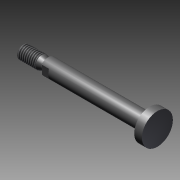
# Autodesk Inventor part: 536203 ADN-15-P-A_(KS)
Saved by Autodesk Inventor 2011 SP1 (Build 150282100, 282)
## iProperties
Created: 2018-05-28
Part Number: 536203 ADN-15-P-A_(KS)
Catalog Web Link: www.cadenas.de
Description: ADN-(KS)-Compact cylinder - piston rod
Vendor: FESTO
Document SubType Name: Modeling
Designer: psAdmin
Manufacturer: FESTO
Mass: 1.6217 g
Surface Area: 12.2965 cm^2
Volume: 1.6217 cm^3
Density: 1 g/cm^3
Category: PARTsolutions
Company: FESTO
Title: 536203 ADN-15-P-A_(KS)
Author: Cadenas PARTsolutions
Comments: Compact cylinder - piston rod
PSOL_IDENT_0: {$CADENAS_DATA\23d-libs\festo\parts\a\adn\parts\adn_ks.prj},229 {VTYP=3D},{NB=536203 ADN-15-P-A_(KS)
PSOL_IDENT_1: },{LINA=536203 ADN-15-P-A_(KS)},{NN=ADN-(KS)},{DATE=06.10.2015 11:54:02},{GEOMDATE=23.09.2015 12:10:
PSOL_IDENT_2: 00},{VERSION=},{LINEID=5510},{LINESUBID=-1},{WBVAR=DF,HUB,TH,Q,S2S20,K2,K5,K8,K10,S1,TT,R8}  {NB=536
PSOL_IDENT_3: 203 ADN-15-P-A_(KS)},{LINA=536203 ADN-15-P-A_(KS)},{KT=536203},{TNR=536203},{AUSF=ADN},{DF=P},{GA=A}
PSOL_IDENT_4: ,{WHX=4.2},{WH0=4.200},{WH1=0.000},{WH2=0.000},{WH3=0.000},{WHX1=4.2},{WHX2=4.75},{WH=4.2},{ZM=44.50
PSOL_IDENT_5: 0},{ZM2=0.000},{ZB=39.200},{ZB1=0.000},{ZB2=0.000},{ZB6=0.000},{ZA=35.000},{KDM=12},{HUBP=-},{HUB=15
PSOL_IDENT_6: },{HUB1=[1-300]},{HUB2=0},{HUB3=0},{HUB4=0},{TH=A},{THC='A','I'},{Q=-},{VAR1C='-','Q'},{S2S20=-},{VA
PSOL_IDENT_7: R2C='-','S2'},{VAR22C='-','S2'},{VAR222C='-','S2'},{K2=0},{VAR3C=0,[1-10]},{VAR33C=0,[1-10]},{K5=-},
PSOL_IDENT_8: {K5A='-','M6'},{K5I='-'},{K5S1A='-'},{K5S1I='-'},{K5C='-','M6'},{K5N=0},{K5P=0},{K5T=},{K8=0},{K10=-
PSOL_IDENT_9: },{K10A='-'},{K10N=},{S1=-},{TT=-},{TT1='-'},{R8=-},{R81='-'},{VAR4C=0,[1-300]},{VAR5C='-','S6'},{VA
PSOL_IDENT_10: R6C='-'},{VAR66C='-'},{VAR7C='-','R3'},{HUBALG=[1-300]},{A=10.000},{A1=0.000},{AF=8.000},{AF1=0.000}
PSOL_IDENT_11: ,{AF2=8.000},{AF3=0.000},{AF5=0.000},{AF7=0.000},{D8=0.000},{D9=0.000},{KF=M3},{KFN=3.000},{KF1=-},{
PSOL_IDENT_12: KF1C=0.0000},{KF2=-},{KF2C=0.0000},{KF3=M3},{KF3C=3.0000},{KF5=-},{KF5N=0},{KF7=-},{KF7N=0},{KK=M5},
PSOL_IDENT_13: {KKN=5},{KKP=0.80},{KK1=-},{KK1N=0.0000},{KK1P=0.00},{L2=35.000},{L8=0.000},{MM=6.000},{MM1=0.000},{
PSOL_IDENT_14: PL=6.000},{SF=5},{SF1=0},{SF3=5.5},{WL=2.700},{WL1=0.000},{QN=},{S2N=},{S1N=},{K2N=},{K8N=},{KKC3=3.
PSOL_IDENT_15: 800},{KKF2=0.400},{KKD5=0.900},{KKE2=20.000},{K5C3=0},{K5F2=0},{K5D5=0},{KK1C3=0.000},{KK1F2=0.000},
PSOL_IDENT_16: {KK1D5=0.000},{KK1E2=0.000},{L100S1=0.000},{L101S1=0.000},{L102S1=0.000},{L103S1=0.000},{D100S1=0.00
PSOL_IDENT_17: 0},{L100=0.400},{L101=1.500},{L102=8.000},{L103=11.000},{D100=3.300},{L100Q=0.400},{L101Q=1.500},{L1
PSOL_IDENT_18: 01K5=1.500},{L102Q=8.000},{L103Q=11.000},{D100Q=3.300},{L100S1K5=0.000},{L101S1K5=0.000},{L102S1K5=0
PSOL_IDENT_19: .000},{L103S1K5=0.000},{D100S1K5=0.000},{VERS=1},{TTN=},{R8N=},{D20=0.000},{XF31=3.000},{B31=2.700},
PSOL_IDENT_20: {DFALG='P'}
NN: ADN-(KS)
NT: Compact cylinder - piston rod
NB: 536203 ADN-15-P-A_(KS)
NBSYN: $TNR. $AUSF.-$HUB.-$DF.-$TH.$QN.$S2N.$K2N.$K5T.$K8N.$K10N.$S1N.$TTN.$R8N._(KS)
LINA: 536203 ADN-15-P-A_(KS)
TNR: 536203
AUSF: ADN
DF: P
GA: A
WHX: 4.200
WH0: 4.200
WH1: 0.000
WH2: 0.000
WH3: 0.000
WHX1: 4.200
WHX2: 4.750
WH: 4.200
ZM: 44.500
ZM2: 0.000
ZB: 39.200
ZB1: 0.000
ZB2: 0.000
ZB6: 0.000
ZA: 35.000
KDM: 12
HUBP: -
HUB: 15
TH: A
Q: -
S2S20: -
K2: 0
K5: -
K8: 0
K10: -
S1: -
TT: -
R8: -
A: 10.000
A1: 0.000
AF: 8.000
AF1: 0.000
AF2: 8.000
AF3: 0.000
AF5: 0.000
AF7: 0.000
D8: 0.000
D9: 0.000
KF: M3
KF1: -
KF2: -
KF3: M3
KF5: -
KF7: -
KK: M5
KK1: -
L2: 35.000
L8: 0.000
MM: 6.000
MM1: 0.000
PL: 6.000
SF: 5
SF1: 0
SF3: 5.5
WL: 2.700
WL1: 0.000
L101K5: 1.500
D20: 0.000
XF31: 3.000
B31: 2.700
SUPPLIER: FESTO
ARTICLENO: 536203 ADN-15-P-A_(KS)
BOMINFO: 536203 ADN-15-P-A_(KS)
CREATOR: CADENAS GmbH
Autodesk Inventor part; units mm, degrees
sketch "Sketch_1" plane through (0, 0, 0) normal (0, 0, 1) x (1, 0, 0)
  line L0 (38, 0) -> (-4.2, 0)
  line L1 (-4.2, 0) -> (-4.2, 3)
  line L2 (-4.2, 3) -> (38, 3)
  line L3 (38, 3) -> (38, 0)
  line L4 (38, 0) -> (-4.2, 0)
  constraints: 10 end point
revolve "Revolution1" add sketch "Sketch_1" angle 360 about axis through (38, 0, 0) along (1, 0, 0)
sketch "Sketch_11" plane through (0, 0, 0) normal (0, 0, 1) x (1, 0, 0)
  line L0 (38, 0) -> (35, 0)
  line L1 (35, 0) -> (35, 6)
  line L2 (35, 6) -> (38, 6)
  line L3 (38, 6) -> (38, 0)
  line L4 (38, 0) -> (35, 0)
  constraints: 10 end point
revolve "Revolution2" add sketch "Sketch_11" angle 360 about axis through (38, 0, 0) along (1, 0, 0)
sketch "Sketch_19" plane through (0, 0, 0) normal (0, 0, 1) x (1, 0, 0)
  line L0 (-3.2, 0) -> (-14.2, 0)
  line L1 (-14.2, 0) -> (-14.2, 2.0095)
  line L2 (-14.2, 2.0095) -> (-13.7095, 2.5)
  line L3 (-13.7095, 2.5) -> (-6.7485, 2.5)
  line L4 (-6.7485, 2.5) -> (-5.1663, 1.9241)
  arc A0 (-5.1663, 1.9241) -> (-5.0295, 1.9) centre (-5.0295, 2.3) ccw
  line L5 (-5.0295, 1.9) -> (-4.6, 1.9)
  arc A1 (-4.6, 1.9) -> (-4.2, 2.3) centre (-4.6, 2.3) ccw
  line L6 (-4.2, 2.3) -> (-4.2, 2.5)
  line L7 (-4.2, 2.5) -> (-3.2, 2.5)
  line L8 (-3.2, 2.5) -> (-3.2, 0)
  line L9 (-3.2, 0) -> (-14.2, 0)
  constraints: 20 end point, 4 point on circle, 2 centre point
revolve "Revolution3" add sketch "Sketch_19" angle 360 about axis through (-3.2, 0, 0) along (1, 0, 0)
thread "Thread1" size "M5x0.8" class "6g" standard "ISO Metric profile" full length
sketch "Sketch_20" plane through (0, 0, 0) normal (0, 0, 1) x (1, 0, 0)
  line L0 (-23.4, -10.5) -> (3.1188, -10.5)
  line L1 (3.1188, -10.5) -> (-1.5, -2.5)
  line L2 (-1.5, -2.5) -> (-4.2, -2.5)
  line L3 (-4.2, -2.5) -> (-4.2, -7.5)
  line L4 (-4.2, -7.5) -> (-19.2, -7.5)
  line L5 (-19.2, -7.5) -> (-19.2, 7.5)
  line L6 (-19.2, 7.5) -> (-4.2, 7.5)
  line L7 (-4.2, 7.5) -> (-4.2, 2.5)
  line L8 (-4.2, 2.5) -> (-1.5, 2.5)
  line L9 (-1.5, 2.5) -> (3.1188, 10.5)
  line L10 (3.1188, 10.5) -> (-23.4, 10.5)
  line L11 (-23.4, 10.5) -> (-23.4, -10.5)
  constraints: 24 end point
extrude "Extrusion1" cut sketch "Sketch_20" along normal mid plane 12
ref_plane "FDT_PIRODACC_M1_XY" through (-9.9, 0, 0) normal (-1, 0, 0) x (0, 1, 0)
ref_plane "FDT_PIRODACC_M1_YZ" through (-9.9, 0, 0) normal (0, 1, 0) x (0, 0, -1)
ref_plane "FDT_PIRODACC_M1_ZX" through (-9.9, 0, 0) normal (0, 0, -1) x (-1, 0, 0)
ref_plane "NUT1_XY" through (-8.55, 0, 0) normal (1, 0, 0) x (0, 0, -1)
ref_plane "NUT1_YZ" through (-8.55, 0, 0) normal (0, 0, -1) x (0, 1, 0)
ref_plane "NUT1_ZX" through (-8.55, 0, 0) normal (0, 1, 0) x (1, 0, 0)
ref_plane "PISTON_XY" through (38, 0, 0) normal (1, 0, 0) x (0, 0, -1)
ref_plane "PISTON_YZ" through (38, 0, 0) normal (0, 0, -1) x (0, 1, 0)
ref_plane "PISTON_ZX" through (38, 0, 0) normal (0, 1, 0) x (1, 0, 0)
body "Solid1"
